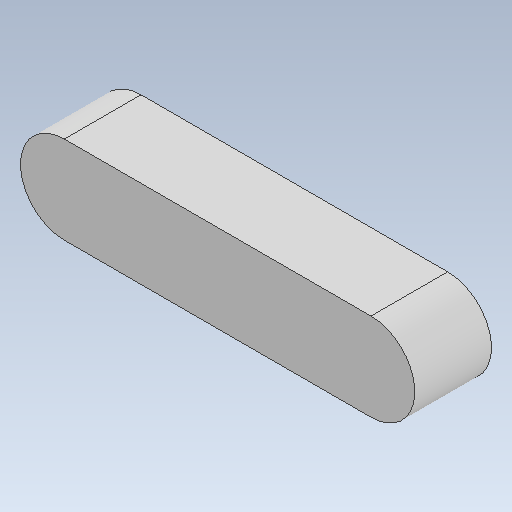
# Autodesk Inventor part: key1
Saved by Autodesk Inventor 2020 (Build 240168000, 168)
## iProperties
Created: 2021-06-15
Part Number: key1
Material: 常规
Document SubType Name: Modeling
Designer: dell
Density: 1 g/cm^3
Appearance: 默认
Author: dell
Autodesk Inventor part; units mm, degrees
ref_plane "YZ Plane" through (0, 0, 0) normal (1, 0, 0) x (0, 1, 0)
ref_plane "XZ Plane" through (0, 0, 0) normal (0, 1, 0) x (-1, 0, 0)
ref_plane "XY Plane" through (0, 0, 0) normal (0, 0, 1) x (1, 0, 0)
sketch "草图1" plane through (0, 0, 0) normal (0, 0, 1) x (1, 0, 0)
  line L0 (-105, 0) -> (-77, 0) projected
  arc A0 (-105, 0) -> (-105, -8) centre (-105, -4) ccw projected
  line L1 (-105, -8) -> (-77, -8) projected
  arc A1 (-77, -8) -> (-77, 0) centre (-77, -4) ccw projected
  line L2 (-105, -4) -> (-77, -4) construction
  line L3 (-105, -8) -> (-77, -8)
  line L4 (-77, 0) -> (-105, 0)
  arc A2 (-105, 0) -> (-105, -8) centre (-105, -4) ccw
  arc A3 (-77, -8) -> (-77, 0) centre (-77, -4) ccw
  point P0 (0, 0)
  point P1 (-91, -4)
  constraints: 8 end point, 4 point on circle, 4 tangent, 2 centre point, 1 concentric, 1 horizontal, 1 midpoint, 1 parallel
extrude "拉伸1" add sketch "草图1" along normal blind 7
